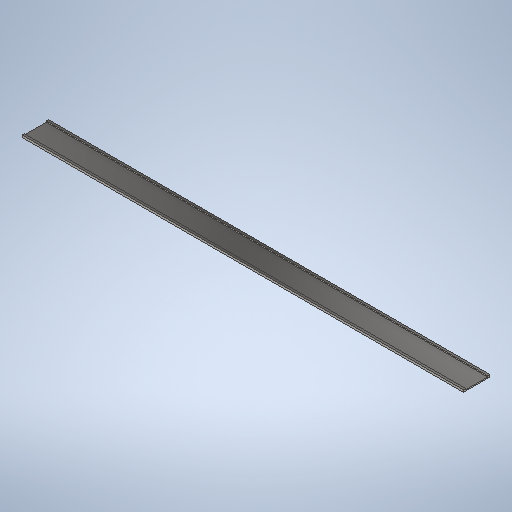
# Autodesk Inventor part: jalur
Saved by Autodesk Inventor 2025 (Build 290162000, 162)
## iProperties
Created: 2024-09-26
Part Number: jalur
Material: Generic
Document SubType Name: Modeling
Designer: DMIADX
Density: 1 g/cm^3
Appearance: Steel - Polished
Author: DMIADX
Autodesk Inventor part; units mm, degrees
ref_plane "YZ Plane" through (0, 0, 0) normal (1, 0, 0) x (0, 1, 0)
ref_plane "XZ Plane" through (0, 0, 0) normal (0, 1, 0) x (-1, 0, 0)
ref_plane "XY Plane" through (0, 0, 0) normal (0, 0, 1) x (1, 0, 0)
sketch "Sketch1" plane through (0, 0, 0) normal (0, 1, 0) x (-1, 0, 0)
  line L0 (-1000, 50) -> (1000, 50)
  line L1 (1000, 50) -> (1000, -50)
  line L2 (1000, -50) -> (-1000, -50)
  line L3 (-1000, -50) -> (-1000, 50)
  line L4 (-1000, 50) -> (1000, -50) construction
  line L5 (1000, 50) -> (-1000, -50) construction
  line L6 (-1000, 60) -> (1000, 60)
  line L7 (1000, 60) -> (1000, -60)
  line L8 (1000, -60) -> (-1000, -60)
  line L9 (-1000, -60) -> (-1000, 60)
  line L10 (-1000, 60) -> (1000, -60) construction
  line L11 (1000, 60) -> (-1000, -60) construction
  point P0 (0, 0)
  dimension "d0" = 100
  dimension "d1" = 2000
  dimension "d2" = 120
  constraints: 24 end point, 4 midpoint, 4 parallel, 2 horizontal, 2 perpendicular, 1 point on line
  measures "d0" distance between parallel lines of L0 L2
  measures "d1" distance of L0.start L0.end
  measures "d2" distance of L6.end L7.end
extrude "Extrusion1" add sketch "Sketch1" against normal blind 5 contours L0 L1 L2 L3
extrude "Extrusion2" add sketch "Sketch1" along normal mid plane 10 contours L9 L6 L7 L0 | L2 L7 L8 L9
body "Solid1"
